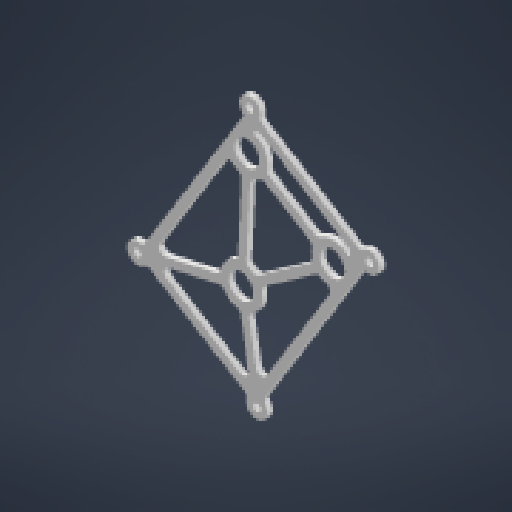
# Autodesk Inventor part: Upper_Plate
Saved by Autodesk Inventor 2024.2 (Build 282272000, 272)
## iProperties
Created: 2024-03-30
Part Number: Upper_Plate
Material: Generic
Document SubType Name: Modeling
Designer: warm
Density: 1 g/cm^3
Appearance: Default
Author: warm
Autodesk Inventor part; units mm, degrees
ref_plane "YZ Plane" through (0, 0, 0) normal (1, 0, 0) x (0, 1, 0)
ref_plane "XZ Plane" through (0, 0, 0) normal (0, 1, 0) x (-1, 0, 0)
ref_plane "XY Plane" through (0, 0, 0) normal (0, 0, 1) x (1, 0, 0)
sketch "Sketch1" plane through (0, 0, 0) normal (0, 0, 1) x (1, 0, 0)
  circle A0 centre (0, 0) radius 7 projected
  circle A1 centre (52.2854, 37.1495) radius 7 projected
  circle A2 centre (3.2487, 67.4218) radius 7 projected
  circle A3 centre (73.2479, 48.3549) radius 2.15
  circle A4 centre (73.9366, 30.5749) radius 3.15 construction
  circle A5 centre (58.8599, 58.8007) radius 3.15 construction
  circle A6 centre (4.7755, 90.6548) radius 2.15
  circle A7 centre (-59.4554, -13.318) radius 2.15
  circle A8 centre (9.0171, -55.618) radius 2.15
  circle A9 centre (38.0853, -27.4589) radius 3.15 construction
  circle A10 centre (-27.4589, -38.0853) radius 3.5 construction
  line L0 (38.0853, -27.4589) -> (9.0171, -55.618) construction
  line L1 (9.0171, -55.618) -> (-27.4589, -38.0853) construction
  line L2 (9.0171, -55.618) -> (73.2479, 48.3549)
  line L3 (92.2333, 46.5881) -> (17.5545, -74.2973) construction
  line L4 (-27.4589, -38.0853) -> (-59.4554, -13.318) construction
  line L5 (-59.4554, -13.318) -> (-42.6755, 23.5008) construction
  line L6 (-59.4554, -13.318) -> (4.7755, 90.6548)
  line L7 (4.7755, 90.6548) -> (73.2479, 48.3549)
  line L8 (9.0171, -55.618) -> (-59.4554, -13.318)
  circle A11 centre (9.0171, -55.618) radius 6
  circle A12 centre (-59.4554, -13.318) radius 6
  circle A13 centre (4.7755, 90.6548) radius 6
  circle A14 centre (73.2479, 48.3549) radius 6
  point P0 (0, 0)
  point P1 (3.9125, -52.4646)
  point P2 (12.1704, -50.5134)
  point P3 (70.0945, 43.2504)
  point P4 (68.1434, 51.5083)
  point P5 (9.88, 87.5015)
  point P6 (1.6221, 85.5503)
  point P7 (-56.302, -8.2135)
  point P8 (-54.3509, -16.4714)
  point P9 (71.4188, 49.4849)
  point P10 (72.118, 46.5258)
  point P11 (3.6455, 88.8257)
  point P12 (6.6046, 89.5249)
  point P13 (-57.6263, -14.448)
  point P14 (-58.3254, -11.4889)
  point P15 (10.147, -53.7888)
  point P16 (7.1879, -54.488)
  dimension "d0" = 4.3
  dimension "d1" = 17.78
  dimension "d2" = 17.78
  dimension "d3" = 4.3
  dimension "d4" = 4.3
  dimension "d5" = 4.3
  dimension "d6" = 40.4622
  dimension "d7" = 12
  dimension "d8" = 12
  dimension "d9" = 12
  dimension "d10" = 12
  constraints: 16 end point, 8 centre point, 4 coincident, 3 parallel, 2 equal length, 1 perpendicular
  measures "d0" diameter of A3
  measures "d1" vertical distance of L2.end A4.centre
  measures "d2" distance of A5.centre L2.end
  measures "d3" diameter of A6
  measures "d4" diameter of A7
  measures "d5" diameter of A8
  measures "d6" distance of L1.end L4.end
  measures "d7" diameter of A11
  measures "d8" diameter of A12
  measures "d9" diameter of A13
  measures "d10" diameter of A14
extrude "Extrusion1" add sketch "Sketch1" along normal blind 3.175 contours A3 L7 A14 L2 | A3 L2 A14 L7 | A14 L2 A11 L8 A12 L6 A13 L7 | A13 L6 A6 L7 | L7 A6 L6 A13 | A11 L8 A8 L2 | L2 A8 L8 A11 | A12 L8 A7 L6 | L6 A7 L8 A12
fillet "Fillet1" radius 3.175 8 edges at (3.9125, -52.4646, 1.5875) (-54.3509, -16.4714, 1.5875) (-56.302, -8.2135, 1.5875) (1.6221, 85.5503, 1.5875) (9.88, 87.5015, 1.5875) (68.1434, 51.5083, 1.5875) (70.0945, 43.2504, 1.5875) (12.1704, -50.5134, 1.5875)
sketch "Sketch2" plane through (0, 0, 0) normal (0, 0, -1) x (-1, 0, 0)
  arc A0 (-13.742, -51.92) -> (-13.5412, -48.2946) centre (-16.2423, -49.9632) ccw projected
  line L0 (-13.5412, -48.2946) -> (-68.7238, 41.0315) projected
  arc A1 (-68.7238, 41.0315) -> (-72.0558, 42.4746) centre (-71.4249, 39.3629) ccw projected
  arc A2 (-69.55, 53.0799) -> (-72.0558, 42.4746) centre (-73.2479, 48.3549) ccw projected
  arc A3 (-69.55, 53.0799) -> (-65.9245, 52.8791) centre (-67.5932, 55.5802) ccw projected
  line L1 (-65.9245, 52.8791) -> (-12.0989, 86.1307) projected
  arc A4 (-12.0989, 86.1307) -> (-10.6559, 89.4627) centre (-13.7676, 88.8318) ccw projected
  arc A5 (-0.0505, 86.9569) -> (-10.6559, 89.4627) centre (-4.7755, 90.6548) ccw projected
  arc A6 (-0.0505, 86.9569) -> (-0.2513, 83.3315) centre (2.4498, 85.0001) ccw projected
  line L2 (-0.2513, 83.3315) -> (54.9312, -5.9946) projected
  arc A7 (54.9312, -5.9946) -> (58.2632, -7.4377) centre (57.6324, -4.326) ccw projected
  arc A8 (55.7575, -18.043) -> (58.2632, -7.4377) centre (59.4554, -13.318) ccw projected
  arc A9 (55.7575, -18.043) -> (52.132, -17.8422) centre (53.8007, -20.5433) ccw projected
  line L3 (52.132, -17.8422) -> (-1.6937, -51.0938) projected
  arc A10 (-1.6937, -51.0938) -> (-3.1367, -54.4258) centre (-0.025, -53.795) ccw projected
  arc A11 (-13.742, -51.92) -> (-3.1367, -54.4258) centre (-9.0171, -55.618) ccw projected
  circle A12 centre (-73.2479, 48.3549) radius 2.15 projected
  circle A13 centre (0, 0) radius 7 projected
  circle A14 centre (-52.2854, 37.1495) radius 7 projected
  circle A15 centre (-3.2487, 67.4218) radius 7 projected
  circle A16 centre (-4.7755, 90.6548) radius 2.15 projected
  circle A17 centre (59.4554, -13.318) radius 2.15 projected
  circle A18 centre (-9.0171, -55.618) radius 2.15 projected
  line L4 (-50.3461, 20.9487) -> (-14.2871, -37.4213)
  arc A19 (-9.7416, -55.0509) -> (-9.2194, -45.6247) centre (-16.2423, -49.9632) ccw
  arc A20 (-9.7416, -55.0509) -> (-8.1154, -55.4352) centre (-9.0171, -55.618) ccw
  arc A21 (-4.3635, -46.772) -> (-8.1154, -55.4352) centre (-0.025, -53.795) ccw
  line L5 (0.8339, -43.5612) -> (42.6394, -17.7352)
  arc A22 (58.8884, -14.0425) -> (49.4621, -13.5204) centre (53.8007, -20.5433) ccw
  arc A23 (58.8884, -14.0425) -> (59.2726, -12.4164) centre (59.4554, -13.318) ccw
  arc A24 (50.6094, -8.6645) -> (59.2726, -12.4164) centre (57.6324, -4.326) ccw
  line L6 (46.6959, -2.3296) -> (9.6075, 57.7068)
  arc A25 (-4.051, 90.0878) -> (-4.5732, 80.6616) centre (2.4498, 85.0001) ccw
  arc A26 (-4.051, 90.0878) -> (-5.6771, 90.4721) centre (-4.7755, 90.6548) ccw
  arc A27 (-9.429, 81.8089) -> (-5.6771, 90.4721) centre (-13.7676, 88.8318) ccw
  line L7 (-11.3353, 80.6312) -> (-60.8723, 50.029)
  arc A28 (-72.6809, 49.0794) -> (-63.2547, 48.5572) centre (-67.5932, 55.5802) ccw
  arc A29 (-72.6809, 49.0794) -> (-73.0651, 47.4533) centre (-73.2479, 48.3549) ccw
  arc A30 (-64.402, 43.7014) -> (-73.0651, 47.4533) centre (-71.4249, 39.3629) ccw
  line L8 (-9.0171, -55.618) -> (0, 0) construction
  line L9 (0, 0) -> (59.4554, -13.318) construction
  line L10 (0, 0) -> (-3.2487, 67.4218) construction
  line L11 (-3.2487, 67.4218) -> (-4.7755, 90.6548) construction
  line L12 (0, 0) -> (-52.2854, 37.1495) construction
  line L13 (-52.2854, 37.1495) -> (-73.2479, 48.3549) construction
  line L14 (-52.2854, 37.1495) -> (-3.2487, 67.4218) construction
  line L15 (-4.7708, -13.5552) -> (-8.4519, -36.2607)
  line L16 (-11.5243, -55.2115) -> (-6.5098, -56.0245) construction
  line L17 (-3.9689, -40.352) -> (0.2437, -14.3682)
  line L18 (2.5073, -0.4065) -> (-2.5073, 0.4065) construction
  line L19 (-2.5073, 0.4065) -> (-6.5098, -56.0245) construction
  line L20 (-11.5243, -55.2115) -> (2.5073, -0.4065) construction
  line L21 (-39.2842, 31.0278) -> (-10.0588, 10.2628)
  line L22 (1.4712, 2.0706) -> (-1.4712, -2.0706) construction
  line L23 (-13.0012, 6.1217) -> (-42.2265, 26.8867)
  line L24 (-53.7566, 35.0789) -> (-50.8142, 39.2201) construction
  line L25 (-50.8142, 39.2201) -> (-1.4712, -2.0706) construction
  line L26 (1.4712, 2.0706) -> (-53.7566, 35.0789) construction
  line L27 (14.3572, -0.6131) -> (43.3008, -7.0964)
  line L28 (60.0106, -10.8395) -> (58.9002, -15.7966) construction
  line L29 (41.6647, -11.9359) -> (13.2468, -5.5702)
  line L30 (-0.5552, -2.4786) -> (0.5552, 2.4786) construction
  line L31 (0.5552, 2.4786) -> (58.9002, -15.7966) construction
  line L32 (60.0106, -10.8395) -> (-0.5552, -2.4786) construction
  line L33 (-3.2178, 14.0054) -> (-5.1051, 53.1719)
  line L34 (-5.7858, 67.2995) -> (-0.7117, 67.544) construction
  line L35 (-0.0309, 53.4164) -> (1.8563, 14.2499)
  line L36 (2.5371, 0.1222) -> (-2.5371, -0.1222) construction
  line L37 (-2.5371, -0.1222) -> (-0.7117, 67.544) construction
  line L38 (-5.7858, 67.2995) -> (2.5371, 0.1222) construction
  line L39 (-13.9498, 57.8305) -> (-38.9157, 42.4181)
  line L40 (-50.9511, 34.9882) -> (-53.6197, 39.3108) construction
  line L41 (-41.5843, 46.7407) -> (-16.6184, 62.1532)
  line L42 (-4.583, 69.5831) -> (-1.9145, 65.2604) construction
  line L43 (-1.9145, 65.2604) -> (-53.6197, 39.3108) construction
  line L44 (-50.9511, 34.9882) -> (-4.583, 69.5831) construction
  line L45 (-63.5617, 46.0573) -> (-60.7004, 44.5278)
  line L46 (-72.0505, 50.595) -> (-74.4453, 46.1149) construction
  line L47 (-74.4453, 46.1149) -> (-53.4828, 34.9094)
  line L48 (-53.4828, 34.9094) -> (-51.088, 39.3895) construction
  line L49 (-51.088, 39.3895) -> (-74.4453, 46.1149) construction
  line L50 (-72.0505, 50.595) -> (-53.4828, 34.9094) construction
  line L51 (-2.241, 90.8214) -> (-0.7142, 67.5883) construction
  line L52 (-0.7142, 67.5883) -> (-5.7833, 67.2552) construction
  line L53 (-6.7107, 81.3688) -> (-6.4984, 78.1383) construction
  line L54 (-7.31, 90.4883) -> (-2.241, 90.8214) construction
  line L55 (-2.241, 90.8214) -> (-5.7833, 67.2552) construction
  line L56 (-0.7142, 67.5883) -> (-7.31, 90.4883) construction
  arc A31 (-3.9689, -40.352) -> (0.8339, -43.5612) centre (-0.8348, -40.8601) ccw
  arc A32 (-14.2871, -37.4213) -> (-8.4519, -36.2607) centre (-11.586, -35.7526) ccw
  arc A33 (42.6394, -17.7352) -> (41.6647, -11.9359) centre (40.9707, -15.0341) ccw
  arc A34 (43.3008, -7.0964) -> (46.6959, -2.3296) centre (43.9948, -3.9982) ccw
  arc A35 (-5.1051, 53.1719) -> (-7.23, 56.0167) centre (-8.2764, 53.0191) ccw
  arc A36 (-8.499, 78.3012) -> (-6.7107, 81.3688) centre (-9.8789, 81.1606) ccw
  arc A37 (-8.499, 78.3012) -> (-15.1565, 65.3891) centre (-3.2487, 67.4218) ccw
  arc A38 (-10.4019, 57.6874) -> (-7.23, 56.0167) centre (-3.2487, 67.4218) ccw
  arc A39 (-10.4019, 57.6874) -> (-13.9498, 57.8305) centre (-12.282, 55.1289) ccw
  arc A40 (-16.6184, 62.1532) -> (-15.1565, 65.3891) centre (-18.2862, 64.8548) ccw
  arc A41 (-6.4984, 78.1383) -> (-11.3353, 80.6312) centre (-9.6666, 77.9301) ccw
  arc A42 (-40.5339, 34.3515) -> (-40.3776, 39.1822) centre (-52.2854, 37.1495) ccw
  arc A43 (-42.2265, 26.8867) -> (-45.7763, 26.9731) centre (-44.0655, 24.2985) ccw
  arc A44 (-45.1322, 46.8839) -> (-60.0296, 46.4206) centre (-52.2854, 37.1495) ccw
  arc A45 (-48.6108, 25.6419) -> (-45.7763, 26.9731) centre (-52.2854, 37.1495) ccw
  arc A46 (-48.6108, 25.6419) -> (-50.3461, 20.9487) centre (-47.645, 22.6174) ccw
  arc A47 (-45.1322, 46.8839) -> (-41.5843, 46.7407) centre (-43.2521, 49.4424) ccw
  arc A48 (-63.5617, 46.0573) -> (-60.0296, 46.4206) centre (-62.065, 48.8574) ccw
  arc A49 (-60.8723, 50.029) -> (-60.7004, 44.5278) centre (-59.2036, 47.3279) ccw
  arc A50 (-40.5339, 34.3515) -> (-39.2842, 31.0278) centre (-37.4452, 33.616) ccw
  arc A51 (-38.9157, 42.4181) -> (-40.3776, 39.1822) centre (-37.2479, 39.7164) ccw
  arc A52 (-5.0594, 10.9695) -> (-6.5091, 10.1764) centre (0, 0) ccw
  arc A53 (-11.7515, 2.798) -> (-6.2597, -10.3317) centre (0, 0) ccw
  arc A54 (2.6748, -11.7802) -> (9.9402, -6.8643) centre (0, 0) ccw
  arc A55 (11.9186, 1.9679) -> (3.9812, 11.4051) centre (0, 0) ccw
  arc A56 (-5.0594, 10.9695) -> (-3.2178, 14.0054) centre (-6.3891, 13.8526) ccw
  arc A57 (-10.0588, 10.2628) -> (-6.5091, 10.1764) centre (-8.2199, 12.851) ccw
  arc A58 (-11.7515, 2.798) -> (-13.0012, 6.1217) centre (-14.8401, 3.5334) ccw
  arc A59 (-4.7708, -13.5552) -> (-6.2597, -10.3317) centre (-7.9049, -13.0471) ccw
  arc A60 (2.6748, -11.7802) -> (0.2437, -14.3682) centre (3.3778, -14.8763) ccw
  arc A61 (13.2468, -5.5702) -> (9.9402, -6.8643) centre (12.5528, -8.6685) ccw
  arc A62 (11.9186, 1.9679) -> (14.3572, -0.6131) centre (15.0512, 2.4851) ccw
  arc A63 (1.8563, 14.2499) -> (3.9812, 11.4051) centre (5.0276, 14.4027) ccw
  arc A64 (1.8106, 56.4523) -> (4.7928, 58.4074) centre (-3.2487, 67.4218) ccw
  arc A65 (1.8106, 56.4523) -> (-0.0309, 53.4164) centre (3.1404, 53.5692) ccw
  arc A66 (9.6075, 57.7068) -> (4.7928, 58.4074) centre (6.9064, 56.0381) ccw
  point P0 (0, 0)
  point P1 (-4.5085, -27.809)
  point P2 (-26.1427, 18.5747)
  point P3 (29.7277, -6.659)
  point P4 (-1.6244, 33.7109)
  point P5 (-27.7671, 52.2856)
  point P6 (-62.7667, 42.7522)
  point P7 (-4.0121, 79.0383)
  point P8 (7.2726, 61.4864)
  point P9 (-52.9015, 25.0852)
  point P10 (-61.9209, 45.6857)
  point P11 (-7.0473, 79.7245)
  dimension "d14" = 5.08
  dimension "d15" = 5.08
  dimension "d16" = 5.08
  dimension "d17" = 5.08
  dimension "d18" = 5.08
  dimension "d19" = 5.08
  dimension "d20" = 5.08
  dimension "d21" = 5.08
  dimension "d22" = 3.175
  dimension "d25" = 3.175
  dimension "d26" = 3.175
  dimension "d27" = 3.175
  dimension "d29" = 3.175
  dimension "d30" = 3.175
  dimension "d31" = 3.175
  dimension "d32" = 3.175
  dimension "d34" = 3.175
  dimension "d35" = 5.08
  dimension "d36" = 3.175
  dimension "d37" = 3.175
  constraints: 106 end point, 98 point on circle, 49 tangent, 48 centre point, 34 point on line, 21 midpoint, 20 parallel, 14 equal radius, 7 perpendicular, 13 other
  measures "d14" distance between parallel lines of L0 L4
  measures "d15" distance of L16.end L16.start
  measures "d16" distance of L22.start L22.end
  measures "d17" distance of L28.start L28.end
  measures "d18" distance of L34.start L34.end
  measures "d19" distance of L40.start L40.end
  measures "d20" distance of L46.end L46.start
  measures "d21" distance of L51.end L52.end
  measures "d22" radius of A31
  measures "d25" radius of A36
  measures "d26" radius of A39
  measures "d27" radius of A41
  measures "d29" radius of A43
  measures "d30" radius of A46
  measures "d31" radius of A48
  measures "d32" radius of A50
  measures "d34" radius of A56
  measures "d35" radial gap between concentric circles of A15 A64
  measures "d36" radius of A65
  measures "d37" radius of A66
extrude "Extrusion2" cut sketch "Sketch2" against normal blind 25.4 contours A46 A45 A43 L23 A58 A53 A59 L15 A32 L4 | A31 L17 A60 A54 A61 L29 A33 L5 | A34 L27 A62 A55 A63 L35 A65 A64 A66 L6 | A41 A36 A37 A40 L41 A47 A44 A48 A49 L7 | A50 A42 A51 L39 A39 A38 A35 L33 A56 A52 A57 L21
body "Solid1"
